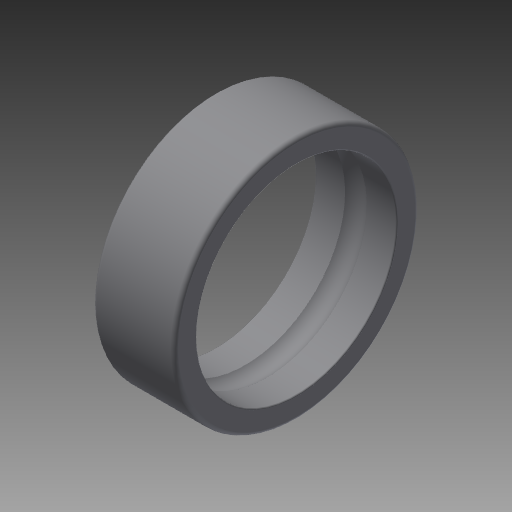
# Autodesk Inventor part: W 617/3_PART2
Saved by Autodesk Inventor 2019.1 (Build 231200000, 200)
## iProperties
Category: PARTsolutions
Company: SKF
Created: 2018-11-24
Part Number: W 617/3_PART2
Material: Allgemein
Catalog Web Link: www.cadenas.de
Description: -Deep groove ball bearings
Vendor: SKF
Document SubType Name: Modeling
Designer: psadmin
Manufacturer: SKF
Mass: 0.0181787 g
Surface Area: 0.86249 cm^2
Volume: 0.0181787 cm^3
Density: 1 g/cm^3
Appearance: PSOLRGB-175-175-175
PSOL_IDENT_0: {$CADENAS_DATA\23d-libs\skf\bearings_units_and_housings\ball_bearings\deep_groove_ball_bearings\bb1_
PSOL_IDENT_1: 001_101.prj},193 {VTYP=3D},{NB=W 617/3_PART2},{LINA=W 617/3_PART2},{NN=BB1_001_101_PART2},{NOPRJ=TRU
PSOL_IDENT_2: E},{DATE=05.11.2018 07:58:23},{GEOMDATE=08.08.2018 12:16:40},{VERSION=},{LINEID=18990},{WBVAR=},{WBN
PSOL_IDENT_3: UMERIC=}  {NB=W 617/3_PART2},{LINA=W 617/3_PART2},{KT=DUMMY},{PRODUCTID=},{DESIGNATION=W 617/3},{DD=
PSOL_IDENT_4: 3.00},{D=6.000},{B=2.000},{C=0.000},{DD1=3.70},{DD2=0.0},{D1=4.90},{D2=0.00},{D3=0.00},{D4=0.000},{H
PSOL_IDENT_5: H=MIN},{BB=0.000},{FF=0.00},{R0MAX=MIN},{R0=MIN},{R12=0.10},{PITCH=4.30},{DW=0.800},{DDAMIN=3.600},{
PSOL_IDENT_6: DDAMAX=MIN},{DDBMIN=MIN},{DDBMAX=MIN},{DBMIN=MIN},{DAMAX=5.200},{BBAMIN=MIN},{CAMAX=MIN},{RAMAX=0.10
PSOL_IDENT_7: 0},{LOAD1=0.117},{LOAD2=0.036},{LOAD3=0.002},{SPEED1=170000},{SPEED2=110000},{KR=0.015},{F0=7.100},{
PSOL_IDENT_8: Z=8},{II=1},{MASS=0.000},{BEARING=W 617/3},{RING=},{HELP=0.550},{HELP2=0.550},{DD1ALG=1.850},{YALG=1
PSOL_IDENT_9: .850},{PITCH1=4.300},{DW1=0.800},{YALG1=2.450},{HALG1=0.550},{SH=1.850},{CU=0.240},{DESIGN=dgbbw},{H
PSOL_IDENT_10: ALG=0.35},{B1=0},{ALGO=1.000}
NT: Deep groove ball bearings
NB: W 617/3_PART2
NBSYN: $DESIGNATION._PART2
LINA: W 617/3_PART2
SUPPLIER: SKF
ARTICLENO: W 617/3_PART2
BOMINFO: W 617/3_PART2
CREATOR: CADENAS GmbH
Title: W 617/3_PART2
Author: Cadenas PARTsolutions
Comments: Deep groove ball bearings
Autodesk Inventor part; units mm, degrees
ref_plane "YZ Plane" through (0, 0, 0) normal (1, 0, 0) x (0, 1, 0)
ref_plane "XZ Plane" through (0, 0, 0) normal (0, 1, 0) x (-1, 0, 0)
ref_plane "XY Plane" through (0, 0, 0) normal (0, 0, 1) x (1, 0, 0)
sketch "Sketch_7" plane through (0, 0, 0) normal (0, 0, 1) x (1, 0, 0)
  line L0 (2, 0) -> (-2, 0)
  arc A0 (0, 2.4833) -> (0.0333, 2.45) centre (0.0333, 2.4833) ccw
  line L1 (0.0333, 2.45) -> (0.7354, 2.45)
  arc A1 (1.2646, 2.45) -> (0.7354, 2.45) centre (1, 2.15) ccw
  line L2 (1.2646, 2.45) -> (1.9667, 2.45)
  arc A2 (1.9667, 2.45) -> (2, 2.4833) centre (1.9667, 2.4833) ccw
  line L3 (2, 2.4833) -> (2, 2.9)
  arc A3 (2, 2.9) -> (1.9, 3) centre (1.9, 2.9) ccw
  line L4 (1.9, 3) -> (0.1, 3)
  arc A4 (0.1, 3) -> (0, 2.9) centre (0.1, 2.9) ccw
  line L5 (0, 2.9) -> (0, 2.4833)
  constraints: 12 end point, 10 point on circle, 5 centre point
revolve "Revolution1" add sketch "Sketch_7" angle 360 about axis through (2, 0, 0) along (1, 0, 0)
body "Solid1"
